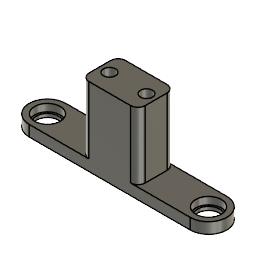
support bridge (Autodesk Fusion 360 design; units mm, degrees)
Autodesk Fusion 360 part; units mm, degrees
note: some values were not read from the file. Set by a fixed rule: which sketch regions a step uses.
sketch "Skizze1" plane through (0, 0, 0) normal (0, 0, 1) x (1, 0, 0)
  line L0 (-22, 5) -> (22, 5)
  line L1 (22, 5) -> (22, -5)
  line L2 (22, -5) -> (-22, -5)
  line L3 (-22, -5) -> (-22, 5)
  circle A0 centre (-22, 0) radius 3.5
  circle A1 centre (22, 0) radius 3.5
  circle A2 centre (-22, 0) radius 5
  circle A3 centre (22, 0) radius 5
  line L4 (-13.5, 5) -> (13.5, 5)
  line L5 (13.5, -5) -> (-13.5, -5)
  circle A4 centre (-22, 0) radius 3
  circle A5 centre (22, 0) radius 3
  circle A6 centre (-5.06, 0) radius 1.65
  circle A7 centre (5.06, 0) radius 1.65
  line L6 (-7.71, 5) -> (7.71, 5)
  line L7 (7.71, -5) -> (-7.71, -5)
  line L8 (-7.71, 5) -> (7.71, 5)
  line L9 (7.71, 5) -> (7.71, -5)
  line L10 (7.71, -5) -> (-7.71, -5)
  line L11 (-7.71, -5) -> (-7.71, 5)
  dimension "d1" = 44
  dimension "d2" = 22
  dimension "d3" = 10
  dimension "d4" = 5
  dimension "d5" = 7
  dimension "d6" = 7
  dimension "d7" = 10
  dimension "d8" = 10
  dimension "d11" = 10
  dimension "d12" = 0
  dimension "d18" = 6
  dimension "d19" = 6
  dimension "d22" = 3.3
  dimension "d23" = 3.3
  dimension "d28" = 10
  dimension "d35" = 15.42
  dimension "d36" = 10
  dimension "d37" = 14.29
  dimension "d40" = 2.65
  dimension "d41" = 2.65
  constraint horizontal L0
  constraint vertical L1
  constraint horizontal L2
  constraint vertical L3
  constraint midpoint L3 A0.centre
  constraint midpoint L1 A1.centre
  constraint concentric A0 A2
  constraint concentric A1 A3
  constraint horizontal L4
  constraint horizontal L5
  constraint concentric A2 A4
  constraint concentric A1 A5
  constraint horizontal L6
  constraint horizontal L7
  constraint collinear L4 L6
  constraint horizontal L8
  constraint vertical L9
  constraint horizontal L10
  constraint vertical L11
  constraint collinear L6 L8
  measures "d1" distance of L1 L3
  measures "d2" distance of origin L1
  measures "d3" distance of L0 L2
  measures "d4" distance of origin L0
  measures "d5" diameter of A0
  measures "d6" diameter of A1
  measures "d7" diameter of A2
  measures "d8" diameter of A3
  measures "d11" distance of L4 L5
  measures "d12" distance of L0 L4
  measures "d18" diameter of A4
  measures "d19" diameter of A5
  measures "d22" diameter of A6
  measures "d23" diameter of A7
  measures "d28" distance of L6 L7
  measures "d35" distance of L9 L11
  measures "d36" distance of L8 L10
  measures "d37" distance of L3 L11
  measures "d40" distance of A7.centre L9
  measures "d41" distance of A6.centre L11
extrude "Extrusion1" add sketch "Skizze1" along normal blind 3 contours L3 A0 A2 | L0 L2 A2 L4 L5 L11 | L3 A0 A2 | L0 L2 L4 L5 L6 L7 L8 L9 L10 L11 | L0 L2 A3 L4 L5 L9 | L1 A1 A3 | L1 A1 A3
extrude "Extrusion3" add sketch "Skizze1" along normal blind 1 contours L3 A0 A4 | L3 A0 A4 | L1 A1 A5 | L1 A1 A5
extrude "Extrusion6" add sketch "Skizze1" along normal blind 18.3 from surface at 3 contours L0 L2 L4 L5 L6 L7 L8 L9 L10 L11
fillet "Abrundung1" radius 2 4 edges at (7.71, 5, 12.15) (-7.71, 5, 12.15) (-7.71, -5, 12.15) (7.71, -5, 12.15)
equation "d2 = d1 / 2"
equation "d4 = d3 / 2"
equation "d6 = d5"
equation "d7 = d3"
equation "d8 = d7"
equation "d11 = d3"
equation "d12 = ( d3 - d11 ) / 2"
equation "d18 = d5 - 1 mm"
equation "d19 = d18"
equation "d23 = d22"
equation "d24 = d31 / 2"
equation "d28 = d11"
equation "d29 = 15.22 mm + 0.2 mm"
equation "d31 = 5.79 mm"
equation "d35 = 15.22 mm + 0.2 mm"
equation "d36 = d11"
equation "d37 = ( d1 - d29 ) / 2"
equation "d40 = d41"
equation "d41 = 1.00 mm + d22 / 2"
equation "d43 = 20.3 mm - 3 mm + 1 mm"
